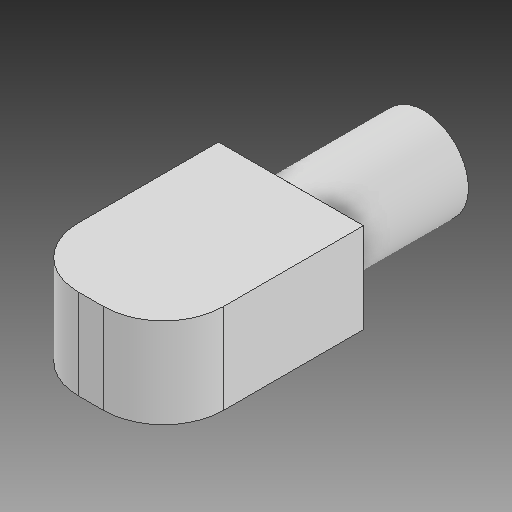
# Autodesk Inventor part: moroshenka
Saved by Autodesk Inventor 2026 (Build 300175000, 175)
## iProperties
Created: 2025-10-18
Part Number: moroshenka
Material: Типовые
Document SubType Name: Modeling
Designer: Admin
Density: 1 g/cm^3
Appearance: По умолчанию
Author: Admin
Autodesk Inventor part; units mm, degrees
ref_plane "YZ Plane" through (0, 0, 0) normal (1, 0, 0) x (0, 1, 0)
ref_plane "XZ Plane" through (0, 0, 0) normal (0, 1, 0) x (-1, 0, 0)
ref_plane "XY Plane" through (0, 0, 0) normal (0, 0, 1) x (1, 0, 0)
sketch "Эскиз1" plane through (0, 0, 0) normal (0, 1, 0) x (-1, 0, 0)
  line L0 (-7.25, -10) -> (7.25, -10)
  line L1 (7.25, -10) -> (7.25, 4)
  line L2 (1.25, 10) -> (-1.25, 10)
  line L3 (-7.25, 4) -> (-7.25, -10)
  line L4 (-7.25, -10) -> (7.25, 10) construction
  line L5 (7.25, -10) -> (-7.25, 10) construction
  arc A0 (7.25, 4) -> (1.25, 10) centre (1.25, 4) ccw
  arc A1 (-1.25, 10) -> (-7.25, 4) centre (-1.25, 4) ccw
  line L6 (0, -10) -> (5, -10)
  point P0 (0, 0)
  dimension "d0" = 14.5
  dimension "d1" = 20
  dimension "d2" = 6
  dimension "d3" = 6
  constraints: 14 end point, 4 point on circle, 4 point on line, 4 tangent, 3 midpoint, 2 centre point, 2 horizontal, 2 parallel, 1 perpendicular
  measures "d0" distance of L5.end L4.end
  measures "d1" distance of L4.end L0.end
  measures "d2" radius of A0
  measures "d3" radius of A1
extrude "Выдавливание1" add sketch "Эскиз1" along normal blind 9
sketch "Эскиз3" plane through (7.25, 0, -10) normal (0, 0, -1) x (-1, 0, 0)
  line L0 (0, 0) -> (0, 9) projected
  line L1 (14.5, 0) -> (8.5, 0) projected
  line L2 (0, 9) -> (14.5, 9)
  line L3 (14.5, 9) -> (14.5, 0)
  line L4 (14.5, 0) -> (0, 0)
  line L5 (0, 0) -> (0, 9)
  circle A0 centre (7, 4.5) radius 4.5
  point P0 (7.25, 0)
  dimension "d11" = 9
  dimension "d12" = 4.5
  constraints: 8 end point, 2 parallel, 1 centre point, 1 horizontal, 1 perpendicular
  measures "d11" diameter of A0
  measures "d12" distance from line of L4 A0.centre
extrude "Выдавливание3" add sketch "Эскиз3" along normal blind 13 contours A0
